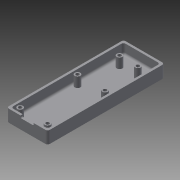
# Autodesk Inventor part: NodeMCU_MQ-4
Saved by Autodesk Inventor 2014 SP1 (Build 180222100, 222)
## iProperties
Created: 2016-10-23
Part Number: NodeMCU_MQ-4
Material: Generic
Document SubType Name: Modeling
Designer: danielsikar
Density: 1 g/cm^3
Appearance: Default
Author: danielsikar
Autodesk Inventor part; units mm, degrees
ref_plane "YZ Plane" through (0, 0, 0) normal (1, 0, 0) x (0, 1, 0)
ref_plane "XZ Plane" through (0, 0, 0) normal (0, 1, 0) x (-1, 0, 0)
ref_plane "XY Plane" through (0, 0, 0) normal (0, 0, 1) x (1, 0, 0)
sketch "Sketch3" plane through (0, 0, 0) normal (0, 0, 1) x (1, 0, 0)
  line L0 (0, 0) -> (37, 0)
  line L1 (37, 0) -> (37, 105.5)
  line L2 (37, 105.5) -> (0, 105.5)
  line L3 (0, 105.5) -> (0, 0)
  dimension "d5" = 37
  dimension "d6" = 105.5
  constraints: 8 end point, 2 parallel, 1 horizontal, 1 perpendicular
  measures "d5" distance of L2.end L1.end
  measures "d6" distance of L1.end L0.end
extrude "Extrusion2" add sketch "Sketch3" along normal blind 2
fillet "Fillet1" radius 2 4 edges at (0, 0, 1) (37, 0, 1) (37, 105.5, 1) (0, 105.5, 1)
sketch "Sketch4" plane through (0, 0, 2) normal (0, 0, 1) x (1, 0, 0)
  arc A0 (2, 105.5) -> (0, 103.5) centre (2, 103.5) ccw projected
  line L0 (0, 103.5) -> (0, 2) projected
  arc A1 (0, 2) -> (2, 0) centre (2, 2) ccw projected
  line L1 (2, 0) -> (35, 0) projected
  arc A2 (35, 0) -> (37, 2) centre (35, 2) ccw projected
  line L2 (37, 2) -> (37, 103.5) projected
  arc A3 (37, 103.5) -> (35, 105.5) centre (35, 103.5) ccw projected
  line L3 (35, 105.5) -> (2, 105.5) projected
  line L4 (2, 0) -> (35, 0)
  line L5 (37, 2) -> (37, 103.5)
  line L6 (35, 105.5) -> (2, 105.5)
  line L7 (0, 103.5) -> (0, 2)
  arc A4 (37, 103.5) -> (35, 105.5) centre (35, 103.5) ccw
  arc A5 (2, 105.5) -> (0, 103.5) centre (2, 103.5) ccw
  arc A6 (0, 2) -> (2, 0) centre (2, 2) ccw
  arc A7 (35, 0) -> (37, 2) centre (35, 2) ccw
  line L8 (35, 101.5) -> (35, 4)
  line L9 (33, 2) -> (4, 2)
  line L10 (2, 4) -> (2, 101.5)
  line L11 (4, 103.5) -> (33, 103.5)
  arc A8 (33, 2) -> (35, 4) centre (33, 4) ccw
  arc A9 (2, 4) -> (4, 2) centre (4, 4) ccw
  arc A10 (4, 103.5) -> (2, 101.5) centre (4, 101.5) ccw
  arc A11 (35, 101.5) -> (33, 103.5) centre (33, 101.5) ccw
  point P0 (0, 0)
  point P1 (37, 105.5)
  point P2 (35, 103.5)
  point P3 (35, 2)
  point P4 (2, 2)
  point P5 (2, 103.5)
  dimension "d10" = 2
  dimension "d11" = 2
  dimension "d12" = 2
  constraints: 16 end point, 16 point on circle, 16 tangent, 13 point on line, 8 centre point, 6 equal radius, 2 parallel, 1 horizontal, 1 perpendicular, 23 other
  measures "d10" radius of A4
  measures "d11" distance between parallel lines of L2 L8
  measures "d12" radius of A8
extrude "Extrusion3" add sketch "Sketch4" along normal blind 9
sketch "Sketch5" plane through (0, 0, 2) normal (0, 0, 1) x (1, 0, 0)
  line L0 (2, 101.5) -> (2, 4) projected
  line L1 (4, 2) -> (33, 2) projected
  circle A0 centre (6.1, 6.1) radius 2.5
  circle A1 centre (6.1, 6.1) radius 1.5
  line L2 (0, 103.5) -> (0, 2) projected
  line L3 (2, 0) -> (35, 0) projected
  circle A2 centre (6.1, 57.9) radius 2.5
  circle A3 centre (6.1, 57.9) radius 1.5
  circle A4 centre (30.9, 6.1) radius 2.5
  circle A5 centre (30.9, 6.1) radius 1.5
  circle A6 centre (30.9, 57.9) radius 2.5
  circle A7 centre (30.9, 57.9) radius 1.5
  circle A8 centre (10.25, 91.7) radius 2.5
  circle A9 centre (10.25, 91.7) radius 1.5
  circle A10 centre (26.75, 91.7) radius 2.5
  circle A11 centre (26.75, 91.7) radius 1.5
  point P0 (0, 0)
  dimension "d15" = 5
  dimension "d16" = 3
  dimension "d17" = 6.1
  dimension "d18" = 6.1
  dimension "d21" = 51.8
  dimension "d24" = 24.8
  dimension "d27" = 5
  dimension "d28" = 33.8
  dimension "d29" = 4.15
  dimension "d30" = 3
  dimension "d31" = 5
  dimension "d32" = 16.5
  dimension "d33" = 3
  constraints: 12 centre point, 6 coincident, 1 horizontal, 1 vertical, 12 other
  measures "d15" diameter of A0
  measures "d16" diameter of A1
  measures "d17" distance from line of A1.centre L2
  measures "d18" distance from line of A0.centre L3
  measures "d21" distance of A0.centre A2.centre
  measures "d24" distance of A0.centre A4.centre
  measures "d27" diameter of A8
  measures "d28" vertical distance of A8.centre A2.centre
  measures "d29" horizontal distance of A8.centre A2.centre
  measures "d30" diameter of A9
  measures "d31" diameter of A10
  measures "d32" distance of A10.centre A8.centre
  measures "d33" diameter of A11
extrude "Extrusion4" add sketch "Sketch5" along normal blind 9
fillet "Fillet2" radius 2 8 edges at (2.5858, 2.5858, 2) (18.5, 2, 2) (34.4142, 2.5858, 2) (35, 52.75, 2) (34.4142, 102.9142, 2) (18.5, 103.5, 2) (2.5858, 102.9142, 2) (2, 52.75, 2)
sketch "Sketch6" plane through (2, 105.5, 0) normal (0, 1, 0) x (1, 0, 0)
  line L0 (33, 0) -> (0, 0) projected
  line L1 (12.5, 0) -> (20.5, 0)
  line L2 (20.5, 0) -> (20.5, -2)
  line L3 (20.5, -2) -> (12.5, -2)
  line L4 (12.5, -2) -> (12.5, 0)
  line L5 (-2, 0) -> (-2, -11) projected
  dimension "d37" = 8
  dimension "d38" = 2
  dimension "d39" = 14.5
  constraints: 8 end point, 2 parallel, 1 horizontal, 1 perpendicular, 1 point on line
  measures "d37" distance of L2.end L3.end
  measures "d38" distance of L1.end L2.end
  measures "d39" distance from line of L3.end L5
extrude "Extrusion5" add sketch "Sketch6" along normal blind 8
fillet "Fillet3" radius 3 4 edges at (22.5, 113.5, 1) (14.5, 113.5, 1) (14.5, 105.5, 1) (22.5, 105.5, 1)
sketch "Sketch7" plane through (11.5, 105.5, 2) normal (0, 0, 1) x (1, 0, 0)
  circle A0 centre (7, 4) radius 1.5
  point P0 (-11.5, -105.5)
  dimension "d43" = 3
  constraints: 1 centre point
  measures "d43" diameter of A0
extrude "Extrusion6" cut sketch "Sketch7" against normal blind 2
sketch "Sketch8" plane through (0, 0, 11) normal (0, 0, 1) x (1, 0, 0)
  line L0 (33, 2) -> (4, 2) projected
  line L1 (2, 0) -> (35, 0) projected
  line L2 (37, 2) -> (37, 103.5) projected
  line L3 (24.5, 0) -> (12.5, 0)
  line L4 (12.5, 0) -> (12.5, 2)
  line L5 (12.5, 2) -> (24.5, 2)
  line L6 (24.5, 2) -> (24.5, 0)
  point P0 (0, 0)
  dimension "d46" = 12
  dimension "d47" = 12.5
  constraints: 8 end point, 2 parallel, 2 point on line, 1 horizontal, 1 perpendicular
  measures "d46" distance of L4.end L5.end
  measures "d47" distance between parallel lines of L6 L2
extrude "Extrusion7" cut sketch "Sketch8" against normal blind 2
fillet "Fillet4" radius 1 2 edges at (12.5, 1, 9) (24.5, 1, 9)
sketch "Sketch9" plane through (0, 0, 2) normal (0, 0, 1) x (1, 0, 0)
  arc A0 (33, 7.4565) -> (29.5435, 4) centre (30.9, 6.1) ccw projected
  arc A1 (33, 59.2565) -> (33, 56.5435) centre (30.9, 57.9) ccw projected
  arc A2 (4, 56.5435) -> (4, 59.2565) centre (6.1, 57.9) ccw projected
  arc A3 (7.4565, 4) -> (4, 7.4565) centre (6.1, 6.1) ccw projected
  circle A4 centre (10.25, 91.7) radius 2.5 projected
  circle A5 centre (26.75, 91.7) radius 2.5 projected
  circle A6 centre (6.1, 57.9) radius 1.5
  circle A7 centre (30.9, 57.9) radius 1.5
  circle A8 centre (26.75, 91.7) radius 1.5
  circle A9 centre (10.25, 91.7) radius 1.5
  circle A10 centre (6.1, 6.1) radius 1.5
  circle A11 centre (30.9, 6.1) radius 1.5
  point P0 (0, 0)
  dimension "d51" = 3
  dimension "d52" = 3
  dimension "d53" = 3
  dimension "d54" = 3
  dimension "d55" = 3
  dimension "d56" = 3
  constraints: 6 centre point, 6 coincident
  measures "d51" diameter of A6
  measures "d52" diameter of A7
  measures "d53" diameter of A8
  measures "d54" diameter of A9
  measures "d55" diameter of A10
  measures "d56" diameter of A11
extrude "Extrusion8" cut sketch "Sketch9" against normal blind 2 contours A6 | A7 | A8 | A9 | A10 | A11
chamfer "Chamfer1" distance 2 angle 45 6 edges at (8.75, 91.7, 0) (25.25, 91.7, 0) (29.4, 57.9, 0) (4.6, 57.9, 0) (29.4, 6.1, 0) (4.6, 6.1, 0)
body "Solid2"
